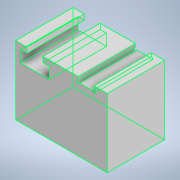
# Autodesk Inventor part: Part1
Saved by Autodesk Inventor 2022 (Build 260153000, 153)
## iProperties
Created: 2022-04-09
Part Number: Part1
Material: Generic
Document SubType Name: Modeling
Designer: Alexandra
Density: 1 g/cm^3
Appearance: Default
Author: Alexandra
Autodesk Inventor part; units mm, degrees
ref_plane "YZ Plane" through (0, 0, 0) normal (1, 0, 0) x (0, 1, 0)
ref_plane "XZ Plane" through (0, 0, 0) normal (0, 1, 0) x (-1, 0, 0)
ref_plane "XY Plane" through (0, 0, 0) normal (0, 0, 1) x (1, 0, 0)
sketch "Sketch1" plane through (0, 0, 0) normal (0, 0, 1) x (1, 0, 0)
  line L0 (-33.6993, 23.1981) -> (46.3007, 23.1981)
  line L1 (46.3007, 23.1981) -> (46.3007, -36.8019)
  line L2 (46.3007, -36.8019) -> (-33.6993, -36.8019)
  line L3 (-33.6993, -36.8019) -> (-33.6993, 23.1981)
  point P0 (0, 0)
  dimension "d0" = 80
  dimension "d1" = 60
  constraints: 8 end point, 2 parallel, 1 horizontal, 1 perpendicular
  measures "d0" distance of L0.start L0.end
  measures "d1" distance of L2.end L0.start
extrude "Extrusion1" add sketch "Sketch1" along normal blind 50
sketch "Sketch2" plane through (0, 0, 50) normal (0, 0, 1) x (1, 0, 0)
  line L0 (-23.918, 27.4616) -> (-23.918, 18.4616)
  line L1 (-23.918, 18.4616) -> (-29.418, 18.4616)
  line L2 (-29.418, 18.4616) -> (-29.418, 8.4616)
  line L3 (-29.418, 8.4616) -> (-4.418, 8.4616)
  line L4 (-4.418, 8.4616) -> (-4.418, 18.4616)
  line L5 (-4.418, 18.4616) -> (-9.918, 18.4616)
  line L6 (-9.918, 18.4616) -> (-9.918, 27.4616)
  line L7 (-9.918, 27.4616) -> (-23.918, 27.4616)
  point P0 (0, 0)
  point P1 (-16.918, 27.4616)
  dimension "d4" = 14
  dimension "d5" = 10
  dimension "d6" = 25
  dimension "d7" = 9
  dimension "d8" = 7
  dimension "d9" = 12.5
  constraints: 16 end point, 6 perpendicular, 2 point on line, 1 midpoint, 1 vertical
  measures "d4" distance of L6.end L0.start
  measures "d5" distance of L1.end L2.end
  measures "d6" distance of L2.end L3.end
  measures "d7" distance of L5.end L6.end
  measures "d8" distance of L0.start point (-16.918, 27.462)
  measures "d9" distance from line of point (-16.918, 27.462) L2
extrude "Extrusion2" cut sketch "Sketch2" against normal blind 50
sketch "Sketch3" plane through (0, 0, 50) normal (0, 0, 1) x (1, 0, 0)
  line L0 (27.8246, 24.0009) -> (34.8246, 24.0009)
  line L1 (34.8246, 24.0009) -> (34.8246, 20.4151)
  line L2 (34.8246, 20.4151) -> (36.2388, 19.0009)
  line L3 (36.2388, 19.0009) -> (34.8246, 17.5867)
  line L4 (34.8246, 17.5867) -> (33.4104, 19.0009)
  line L5 (33.4104, 19.0009) -> (27.8246, 19.0009)
  line L6 (27.8246, 24.0009) -> (27.8246, 19.0009) construction
  line L7 (27.8246, 24.0009) -> (20.8246, 24.0009)
  line L8 (20.8246, 24.0009) -> (20.8246, 20.4151)
  line L9 (20.8246, 20.4151) -> (19.4104, 19.0009)
  line L10 (19.4104, 19.0009) -> (20.8246, 17.5867)
  line L11 (20.8246, 17.5867) -> (22.2388, 19.0009)
  line L12 (22.2388, 19.0009) -> (27.8246, 19.0009)
  point P0 (0, 0)
  dimension "d12" = 2
  dimension "d13" = 7
  dimension "d14" = 5
  dimension "d15" = 135
  dimension "d16" = 2
  constraints: 26 end point, 5 symmetric about line, 3 perpendicular, 2 parallel, 1 coincident, 1 horizontal, 1 vertical
  measures "d12" distance of L1.end L2.end
  measures "d13" distance of L0.start L0.end
  measures "d14" distance of L6.start L5.end
  measures "d15" angle of L5 L4
  measures "d16" distance of L2.end L3.end
extrude "Extrusion3" cut sketch "Sketch3" against normal blind 50
body "Solid1"
